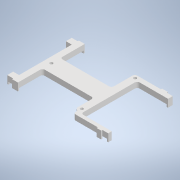
# Autodesk Inventor part: display_holder
Saved by Autodesk Inventor 2022 (Build 260153000, 153)
## iProperties
Created: 2021-12-06
Part Number: display_holder
Material: Generic
Document SubType Name: Modeling
Designer: simen
Density: 1 g/cm^3
Appearance: Default
Author: simen
## iProperties of the stored document display_holder_3DPrint.ipt
Created: 2021-12-08
Part Number: display_holder_3DPrint
Material: Generic
Document SubType Name: Modeling
Designer: simen
Density: 1 g/cm^3
Appearance: Default
Author: simen
Autodesk Inventor part; units mm, degrees
ref_plane "YZ Plane" through (0, 0, 0) normal (1, 0, 0) x (0, 1, 0)
ref_plane "XZ Plane" through (0, 0, 0) normal (0, 1, 0) x (-1, 0, 0)
ref_plane "XY Plane" through (0, 0, 0) normal (0, 0, 1) x (1, 0, 0)
sketch "Sketch9" plane through (0, 0, 0) normal (0, 1, 0) x (-1, 0, 0)
  line L0 (80.3, -1) -> (75.3, -1)
  line L1 (75.3, -1) -> (75.3, 0)
  line L2 (75.3, 0) -> (70.3, 0)
  line L3 (70.3, 0) -> (70.3, -18.75)
  line L4 (68.3, -20.75) -> (29, -20.75)
  line L5 (0, 0) -> (0, -1)
  line L6 (0, -1) -> (-5, -1)
  line L7 (-5, -1) -> (-5, -4)
  line L8 (-5, -4) -> (19, -4)
  line L9 (21, -6) -> (21, -49.5)
  line L10 (19, -51.5) -> (-5, -51.5)
  line L11 (-5, -51.5) -> (-5, -55.5)
  line L12 (-5, -55.5) -> (0, -55.5)
  line L13 (29, -35.75) -> (68.3, -35.75)
  line L14 (70.3, -37.75) -> (70.3, -56.5)
  line L15 (70.3, -56.5) -> (75.3, -56.5)
  line L16 (75.3, -56.5) -> (75.3, -55.5)
  line L17 (75.3, -55.5) -> (80.3, -55.5)
  line L18 (80.3, -55.5) -> (80.3, -50.5)
  line L19 (80.3, -50.5) -> (75.3, -50.5)
  line L20 (75.3, -50.5) -> (75.3, -6)
  line L21 (75.3, -6) -> (80.3, -6)
  line L22 (80.3, -6) -> (80.3, -1)
  line L23 (27, -37.75) -> (27, -53.5)
  line L24 (25, -55.5) -> (5, -55.5)
  line L25 (0, -55.5) -> (0, -56.5)
  line L26 (0, -56.5) -> (5, -56.5)
  line L27 (5, -56.5) -> (5, -55.5)
  line L28 (3.9072, 0) -> (3.9072, -1)
  line L29 (3.9072, -1) -> (25, -1)
  line L30 (27, -3) -> (27, -18.75)
  line L31 (3.9072, 0) -> (0, 0)
  arc A0 (19, -51.5) -> (21, -49.5) centre (19, -49.5) ccw
  arc A1 (21, -6) -> (19, -4) centre (19, -6) ccw
  arc A2 (27, -3) -> (25, -1) centre (25, -3) ccw
  arc A3 (25, -55.5) -> (27, -53.5) centre (25, -53.5) ccw
  arc A4 (70.3, -37.75) -> (68.3, -35.75) centre (68.3, -37.75) ccw
  arc A5 (68.3, -20.75) -> (70.3, -18.75) centre (68.3, -18.75) ccw
  arc A6 (29, -35.75) -> (27, -37.75) centre (29, -37.75) ccw
  arc A7 (27, -18.75) -> (29, -20.75) centre (29, -18.75) ccw
  point P0 (70.3, -20.75)
  point P1 (27, -20.75)
  point P2 (21, -4)
  point P3 (21, -51.5)
  point P4 (27, -35.75)
  point P5 (70.3, -35.75)
  point P6 (27, -55.5)
  point P7 (27, -1)
  dimension "d42" = 85.3
  dimension "d45" = 15
  dimension "d46" = 5
  dimension "d47" = 5
  dimension "d48" = 5
  dimension "d50" = 1
  dimension "d60" = 4
  dimension "d62" = 26
  dimension "d64" = 1
  dimension "d65" = 5
  dimension "d66" = 5
  dimension "d67" = 6
  dimension "d68" = 3
  dimension "d69" = 56.5
  dimension "d70" = 5
  dimension "d90" = 2
  dimension "d91" = 2
  dimension "d92" = 2
  constraints: 64 end point, 21 point on line, 20 perpendicular, 16 point on circle, 16 tangent, 11 collinear, 8 centre point, 5 equal radius, 3 vertical, 1 coincident, 1 horizontal, 1 parallel
  measures "d42" distance between parallel lines of L18 L11
  measures "d45" distance between parallel lines of L13 L4
  measures "d46" distance of L0.start L0.end
  measures "d47" distance of L5.end L6.end
  measures "d48" distance of L1.end L2.end
  measures "d50" distance of L0.end L1.end
  measures "d60" distance of L10.end L11.end
  measures "d62" distance between parallel lines of L9 L11
  measures "d64" distance of L12.end L25.end
  measures "d65" distance of L25.end L26.end
  measures "d66" distance of L11.end L12.end
  measures "d67" distance between parallel lines of L23 L9
  measures "d68" distance of L6.end L7.end
  measures "d69" distance between parallel lines of L31 L26
  measures "d70" distance of L21.end L0.start
  measures "d90" radius of A0
  measures "d91" radius of A4
  measures "d92" radius of A6
extrude "Extrusion9" add sketch "Sketch9" along normal blind 4.5
sketch "Sketch10" plane through (0, 4.5, 0) normal (0, 1, 0) x (1, 0, 0)
  line L0 (-19, 51.5) -> (5, 51.5) projected
  line L1 (0, 0) -> (0, 1) projected
  line L2 (0, 55.5) -> (0, 56.5) projected
  line L3 (5, 55.5) -> (0, 55.5) projected
  line L4 (5, 51.5) -> (5, 55.5) projected
  line L5 (-70.3, 37.75) -> (-70.3, 56.5) projected
  line L6 (-70.3, 56.5) -> (-75.3, 56.5) projected
  line L7 (-75.3, 56.5) -> (-75.3, 55.5) projected
  line L8 (-75.3, 55.5) -> (-80.3, 55.5) projected
  line L9 (-80.3, 55.5) -> (-80.3, 50.5) projected
  line L10 (-80.3, 50.5) -> (-75.3, 50.5) projected
  line L11 (-75.3, 50.5) -> (-75.3, 6) projected
  line L12 (-75.3, 6) -> (-80.3, 6) projected
  line L13 (-80.3, 6) -> (-80.3, 1) projected
  line L14 (-80.3, 1) -> (-75.3, 1) projected
  line L15 (-75.3, 1) -> (-75.3, 0) projected
  line L16 (-75.3, 0) -> (-70.3, 0) projected
  line L17 (-70.3, 0) -> (-70.3, 18.75) projected
  line L18 (-68.3, 20.75) -> (-29, 20.75) projected
  line L19 (-27, 18.75) -> (-27, 3) projected
  line L20 (-25, 1) -> (-3.9072, 1) projected
  line L21 (-3.9072, 1) -> (-3.9072, 0) projected
  line L22 (-3.9072, 0) -> (0, 0) projected
  line L23 (0, 0) -> (0, 1) projected
  line L24 (0, 1) -> (5, 1) projected
  line L25 (5, 1) -> (5, 4) projected
  line L26 (5, 4) -> (-19, 4) projected
  line L27 (-21, 6) -> (-21, 49.5) projected
  line L28 (-19, 51.5) -> (5, 51.5) projected
  line L29 (5, 51.5) -> (5, 55.5) projected
  line L30 (5, 55.5) -> (0, 55.5) projected
  line L31 (0, 55.5) -> (0, 56.5) projected
  line L32 (0, 56.5) -> (-5, 56.5) projected
  line L33 (-5, 56.5) -> (-5, 55.5) projected
  line L34 (-5, 55.5) -> (-25, 55.5) projected
  line L35 (-27, 53.5) -> (-27, 37.75) projected
  line L36 (-29, 35.75) -> (-68.3, 35.75) projected
  line L37 (-27, 1) -> (-3.9072, 1) projected
  line L38 (0, 1) -> (-3.9072, 1)
  line L39 (0, 1) -> (5, 1) projected
  line L40 (4, 1) -> (4, 4)
  line L41 (5, 4) -> (-21, 4) projected
  line L42 (4, 51.5) -> (4, 55.5)
  line L43 (-5, 55.5) -> (-27, 55.5) projected
  line L44 (0, 55.5) -> (-5, 55.5)
  line L45 (-75.3, 55.5) -> (-80.3, 55.5) projected
  line L46 (-75.3, 55.5) -> (-70.3, 55.5)
  line L47 (-80.3, 1) -> (-75.3, 1) projected
  line L48 (-79.3, 1) -> (-79.3, 6)
  line L49 (-75.3, 1) -> (-70.3, 1)
  line L50 (-70.3, 0) -> (-70.3, 20.75) projected
  line L51 (-80.3, 50.5) -> (-75.3, 50.5) projected
  line L52 (-79.3, 50.5) -> (-79.3, 55.5)
  arc A0 (-68.3, 20.75) -> (-70.3, 18.75) centre (-68.3, 18.75) ccw projected
  arc A1 (-27, 18.75) -> (-29, 20.75) centre (-29, 18.75) ccw projected
  arc A2 (-27, 3) -> (-25, 1) centre (-25, 3) ccw projected
  arc A3 (-21, 6) -> (-19, 4) centre (-19, 6) ccw projected
  arc A4 (-19, 51.5) -> (-21, 49.5) centre (-19, 49.5) ccw projected
  arc A5 (-25, 55.5) -> (-27, 53.5) centre (-25, 53.5) ccw projected
  arc A6 (-29, 35.75) -> (-27, 37.75) centre (-29, 37.75) ccw projected
  arc A7 (-70.3, 37.75) -> (-68.3, 35.75) centre (-68.3, 37.75) ccw projected
  point P0 (-75.3, 1)
  dimension "d71" = 1
  dimension "d72" = 1
  dimension "d73" = 1
  dimension "d74" = 1
  constraints: 16 end point, 8 point on line, 3 horizontal, 3 perpendicular, 1 collinear, 1 vertical, 2 other
  measures "d71" distance between parallel lines of L13 L48
  measures "d72" distance between parallel lines of L9 L52
  measures "d73" distance between parallel lines of L4 L42
  measures "d74" distance between parallel lines of L25 L40
extrude "Extrusion10" add sketch "Sketch10" against normal blind 6.5 contours L42 L3 L4 L0 | L44 L33 L32 L2 | L26 L25 L24 L40 | L1 L22 L21 L38 | L46 L7 L6 L5 | L52 L10 L9 L8 | L17 L16 L15 L49 | L14 L13 L12 L48
sketch "Sketch11" plane through (0, 4.5, 0) normal (0, 1, 0) x (1, 0, 0)
  line L0 (5, 4) -> (-19, 4) projected
  line L1 (-21, 6) -> (-21, 49.5) projected
  line L2 (-19, 51.5) -> (5, 51.5) projected
  line L3 (5, 51.5) -> (5, 55.5) projected
  line L4 (5, 55.5) -> (0, 55.5) projected
  line L5 (0, 55.5) -> (0, 56.5) projected
  line L6 (0, 56.5) -> (-5, 56.5) projected
  line L7 (-5, 56.5) -> (-5, 55.5) projected
  line L8 (-5, 55.5) -> (-25, 55.5) projected
  line L9 (-27, 53.5) -> (-27, 37.75) projected
  line L10 (-29, 35.75) -> (-68.3, 35.75) projected
  line L11 (-70.3, 37.75) -> (-70.3, 56.5) projected
  line L12 (-70.3, 56.5) -> (-75.3, 56.5) projected
  line L13 (-75.3, 56.5) -> (-75.3, 55.5) projected
  line L14 (-75.3, 55.5) -> (-80.3, 55.5) projected
  line L15 (-80.3, 55.5) -> (-80.3, 50.5) projected
  line L16 (-80.3, 50.5) -> (-75.3, 50.5) projected
  line L17 (-75.3, 50.5) -> (-75.3, 6) projected
  line L18 (-75.3, 6) -> (-80.3, 6) projected
  line L19 (-80.3, 6) -> (-80.3, 1) projected
  line L20 (-80.3, 1) -> (-75.3, 1) projected
  line L21 (-75.3, 1) -> (-75.3, 0) projected
  line L22 (-75.3, 0) -> (-70.3, 0) projected
  line L23 (-70.3, 0) -> (-70.3, 18.75) projected
  line L24 (-68.3, 20.75) -> (-29, 20.75) projected
  line L25 (-27, 18.75) -> (-27, 3) projected
  line L26 (-25, 1) -> (-3.9072, 1) projected
  line L27 (-3.9072, 1) -> (-3.9072, 0) projected
  line L28 (-3.9072, 0) -> (0, 0) projected
  line L29 (0, 0) -> (0, 1) projected
  line L30 (0, 1) -> (5, 1) projected
  line L31 (5, 1) -> (5, 4) projected
  circle A0 centre (-70.3, 28.25) radius 1.25
  line L32 (-21, 4) -> (-21, 49.5) projected
  line L33 (-75.3, 50.5) -> (-75.3, 6) projected
  arc A1 (-21, 6) -> (-19, 4) centre (-19, 6) ccw projected
  arc A2 (-19, 51.5) -> (-21, 49.5) centre (-19, 49.5) ccw projected
  arc A3 (-25, 55.5) -> (-27, 53.5) centre (-25, 53.5) ccw projected
  arc A4 (-29, 35.75) -> (-27, 37.75) centre (-29, 37.75) ccw projected
  arc A5 (-70.3, 37.75) -> (-68.3, 35.75) centre (-68.3, 37.75) ccw projected
  arc A6 (-68.3, 20.75) -> (-70.3, 18.75) centre (-68.3, 18.75) ccw projected
  arc A7 (-27, 18.75) -> (-29, 20.75) centre (-29, 18.75) ccw projected
  arc A8 (-27, 3) -> (-25, 1) centre (-25, 3) ccw projected
  circle A9 centre (-24.1, 7.75) radius 1.25
  circle A10 centre (-24.1, 52.75) radius 1.25
  line L34 (4, 4) -> (4, 1) projected
  line L35 (0, 1) -> (4, 1) projected
  line L36 (0, 1) -> (-3.9072, 1) projected
  line L37 (-25, 1) -> (-3.9072, 1) projected
  arc A11 (-27, 3) -> (-25, 1) centre (-25, 3) ccw projected
  line L38 (-27, 18.75) -> (-27, 3) projected
  arc A12 (-27, 18.75) -> (-29, 20.75) centre (-29, 18.75) ccw projected
  line L39 (-68.3, 20.75) -> (-29, 20.75) projected
  arc A13 (-68.3, 20.75) -> (-70.3, 18.75) centre (-68.3, 18.75) ccw projected
  line L40 (-70.3, 1) -> (-70.3, 18.75) projected
  line L41 (-70.3, 1) -> (-75.3, 1) projected
  line L42 (-79.3, 1) -> (-75.3, 1) projected
  line L43 (-79.3, 1) -> (-79.3, 6) projected
  line L44 (-75.3, 6) -> (-79.3, 6) projected
  line L45 (-75.3, 50.5) -> (-75.3, 6) projected
  line L46 (-79.3, 50.5) -> (-75.3, 50.5) projected
  line L47 (-79.3, 50.5) -> (-79.3, 55.5) projected
  line L48 (-75.3, 55.5) -> (-79.3, 55.5) projected
  line L49 (-75.3, 55.5) -> (-70.3, 55.5) projected
  line L50 (-70.3, 37.75) -> (-70.3, 55.5) projected
  arc A14 (-70.3, 37.75) -> (-68.3, 35.75) centre (-68.3, 37.75) ccw projected
  line L51 (-29, 35.75) -> (-68.3, 35.75) projected
  arc A15 (-29, 35.75) -> (-27, 37.75) centre (-29, 37.75) ccw projected
  line L52 (-27, 53.5) -> (-27, 37.75) projected
  arc A16 (-25, 55.5) -> (-27, 53.5) centre (-25, 53.5) ccw projected
  line L53 (-5, 55.5) -> (-25, 55.5) projected
  line L54 (-5, 55.5) -> (0, 55.5) projected
  line L55 (4, 55.5) -> (0, 55.5) projected
  line L56 (4, 55.5) -> (4, 51.5) projected
  line L57 (-19, 51.5) -> (4, 51.5) projected
  arc A17 (-19, 51.5) -> (-21, 49.5) centre (-19, 49.5) ccw projected
  line L58 (-21, 6) -> (-21, 49.5) projected
  arc A18 (-21, 6) -> (-19, 4) centre (-19, 6) ccw projected
  line L59 (4, 4) -> (-19, 4) projected
  dimension "d76" = 2.5
  dimension "d93" = 2.5
  dimension "d94" = 2.5
  dimension "d96" = 56.2
  dimension "d97" = 56.2
  dimension "d100" = 7.5
  dimension "d101" = 17
  dimension "d102" = 13
  constraints: 3 centre point, 1 point on line
  measures "d76" diameter of A0
  measures "d93" diameter of A10
  measures "d94" diameter of A9
  measures "d96" distance from line of L19 A9.centre
  measures "d97" distance from line of L15 A10.centre
  measures "d100" distance from line of L10 A0.centre
  measures "d101" distance from line of L10 A10.centre
  measures "d102" distance from line of L24 A9.centre
extrude "Extrusion11" cut sketch "Sketch11" against normal through all contours A0 | A9 | A10
sketch "Sketch14" plane through (0, 0, 0) normal (0, -1, 0) x (1, 0, 0)
  circle A0 centre (-70.3, -28.25) radius 1.25 projected
  circle A1 centre (-24.1, -52.75) radius 1.25 projected
  circle A2 centre (-24.1, -7.75) radius 1.25 projected
  line L0 (4, -4) -> (4, -1) projected
  line L1 (0, -1) -> (4, -1) projected
  line L2 (0, -1) -> (-3.9072, -1) projected
  line L3 (-25, -1) -> (-3.9072, -1) projected
  arc A3 (-25, -1) -> (-27, -3) centre (-25, -3) ccw projected
  line L4 (-27, -18.75) -> (-27, -3) projected
  arc A4 (-29, -20.75) -> (-27, -18.75) centre (-29, -18.75) ccw projected
  line L5 (-68.3, -20.75) -> (-29, -20.75) projected
  arc A5 (-70.3, -18.75) -> (-68.3, -20.75) centre (-68.3, -18.75) ccw projected
  line L6 (-70.3, -1) -> (-70.3, -18.75) projected
  line L7 (-70.3, -1) -> (-75.3, -1) projected
  line L8 (-79.3, -1) -> (-75.3, -1) projected
  line L9 (-79.3, -1) -> (-79.3, -6) projected
  line L10 (-75.3, -6) -> (-79.3, -6) projected
  line L11 (-75.3, -50.5) -> (-75.3, -6) projected
  line L12 (-79.3, -50.5) -> (-75.3, -50.5) projected
  line L13 (-79.3, -50.5) -> (-79.3, -55.5) projected
  line L14 (-75.3, -55.5) -> (-79.3, -55.5) projected
  line L15 (-75.3, -55.5) -> (-70.3, -55.5) projected
  line L16 (-70.3, -37.75) -> (-70.3, -55.5) projected
  arc A6 (-68.3, -35.75) -> (-70.3, -37.75) centre (-68.3, -37.75) ccw projected
  line L17 (-29, -35.75) -> (-68.3, -35.75) projected
  arc A7 (-27, -37.75) -> (-29, -35.75) centre (-29, -37.75) ccw projected
  line L18 (-27, -53.5) -> (-27, -37.75) projected
  arc A8 (-27, -53.5) -> (-25, -55.5) centre (-25, -53.5) ccw projected
  line L19 (-5, -55.5) -> (-25, -55.5) projected
  line L20 (-5, -55.5) -> (0, -55.5) projected
  line L21 (4, -55.5) -> (0, -55.5) projected
  line L22 (4, -55.5) -> (4, -51.5) projected
  line L23 (-19, -51.5) -> (4, -51.5) projected
  arc A9 (-21, -49.5) -> (-19, -51.5) centre (-19, -49.5) ccw projected
  line L24 (-21, -6) -> (-21, -49.5) projected
  arc A10 (-19, -4) -> (-21, -6) centre (-19, -6) ccw projected
  line L25 (4, -4) -> (-19, -4) projected
  line L26 (-27, -18.75) -> (-27, -3) projected
  line L27 (-25, -1) -> (-3.9072, -1) projected
  line L28 (-27, -5.5) -> (-26.5, -5.5)
  line L29 (-24.5, -3.5) -> (-24.5, -1)
  line L30 (-24.5, -1) -> (-27, -1)
  line L31 (-27, -1) -> (-27, -5.5)
  arc A11 (-26.5, -5.5) -> (-24.5, -3.5) centre (-26.5, -3.5) ccw
  point P0 (0, 0)
  dimension "d103" = 2
  dimension "d104" = 4.5
  dimension "d105" = 2.5
  constraints: 8 end point, 2 parallel, 2 point on circle, 2 point on line, 2 tangent, 1 centre point, 1 horizontal, 1 perpendicular
  measures "d103" radius of A11
  measures "d104" distance of L30.end L28.start
  measures "d105" distance of L29.end L30.end
extrude "Extrusion14" cut sketch "Sketch14" against normal through all contours L29 A11 L28 L4 A3 L3
fillet "Fillet1" radius 2 2 edges at (-27, 2.25, -5.5) (-24.5, 2.25, -1)
body "Solid3"
